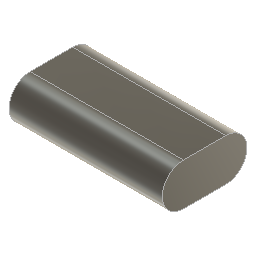
LiPo_Bat_4400_Dual_Cylinder (Autodesk Fusion 360 design; units mm, degrees)
Autodesk Fusion 360 part; units mm, degrees
sketch "Sketch1" plane through (0, 0, 0) normal (0, 0, 1) x (1, 0, 0) in component "LiPo_Bat_4400_Dual_Cylinder"
  line L0 (33.5, 18.5) -> (-33.5, 18.5)
  line L1 (-33.5, 18.5) -> (-33.5, -18.5)
  line L2 (-33.5, -18.5) -> (33.5, -18.5)
  line L3 (33.5, -18.5) -> (33.5, 18.5)
  line L4 (33.5, 18.5) -> (-33.5, -18.5) construction
  line L5 (-33.5, 18.5) -> (33.5, -18.5) construction
  dimension "d1" = 67
  dimension "d2" = 37
  constraint horizontal L0
  constraint perpendicular L0 L1
  constraint parallel L0 L2
  constraint parallel L1 L3
  constraint coincident L4 origin
  constraint coincident L5 origin
  measures "d1" distance of L1.end L2.end
  measures "d2" distance of L0.end L1.end
extrude "Extrude1" add sketch "Sketch1" along normal blind 18.5 in component "LiPo_Bat_4400_Dual_Cylinder"
fillet "Fillet1" radius 9.25 4 edges at (0, -18.5, 18.5) (0, -18.5, 0) (0, 18.5, 0) (0, 18.5, 18.5) in component "LiPo_Bat_4400_Dual_Cylinder"
component "LiPo_Bat_4400_Dual_Cylinder" placed x (1, 0, 0) y (0, 1, 0) z (0, 0, 1) at (0, 0, 0)
